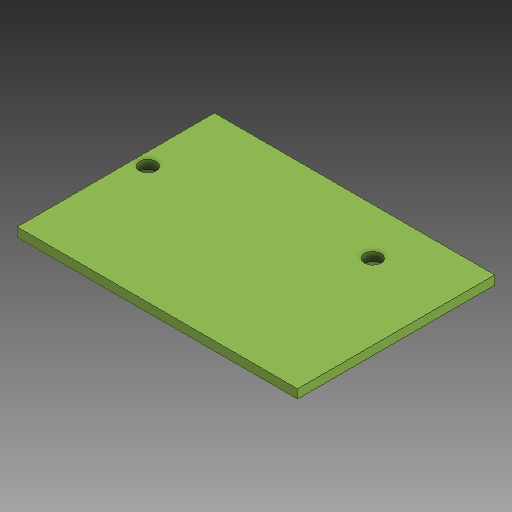
# Autodesk Inventor part: mega_switchboard
Saved by Autodesk Inventor 2020 (Build 240168000, 168)
## iProperties
Created: 2024-09-19
Part Number: mega_switchboard
Material: Типовые
Document SubType Name: Modeling
Designer: Ivan
Density: 1 g/cm^3
Appearance: Оливково-зеленый
Author: Ivan
Autodesk Inventor part; units mm, degrees
ref_plane "YZ Plane" through (0, 0, 0) normal (1, 0, 0) x (0, 1, 0)
ref_plane "XZ Plane" through (0, 0, 0) normal (0, 1, 0) x (-1, 0, 0)
ref_plane "XY Plane" through (0, 0, 0) normal (0, 0, 1) x (1, 0, 0)
sketch "Эскиз1" plane through (0, 0, 0) normal (0, 1, 0) x (-1, 0, 0)
  circle A0 centre (-4.9268, 7.9299) radius 1.6
  line L0 (-19.4268, -1.0701) -> (34.5732, -1.0701)
  line L1 (34.5732, -1.0701) -> (34.5732, 36.9299)
  line L2 (34.5732, 36.9299) -> (-19.4268, 36.9299)
  line L3 (-19.4268, 36.9299) -> (-19.4268, -1.0701)
  circle A1 centre (32.1091, 14.2199) radius 1.6
  point P0 (0, 0)
  constraints: 8 end point, 2 centre point, 2 parallel, 1 horizontal, 1 perpendicular
extrude "Выдавливание1" add sketch "Эскиз1" along normal blind 1.7
